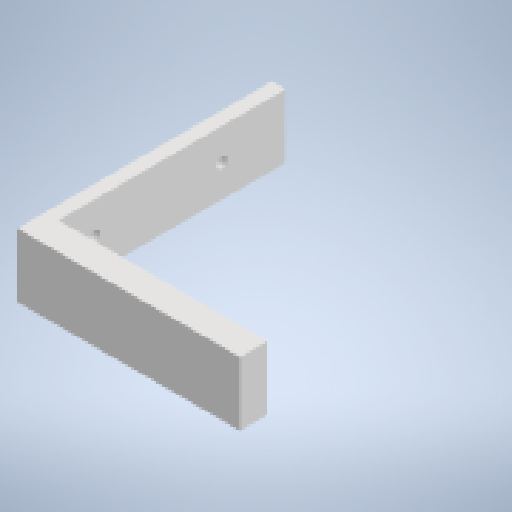
# Autodesk Inventor part: battery shim
Saved by Autodesk Inventor 2023 (Build 270158000, 158)
## iProperties
Created: 2023-02-08
Part Number: battery shim
Material: Generic
Document SubType Name: Modeling
Designer: Gabriel - T3 CAD
Density: 1 g/cm^3
Appearance: Default
Author: Gabriel - T3 CAD
Autodesk Inventor part; units mm, degrees
ref_plane "YZ Plane" through (0, 0, 0) normal (1, 0, 0) x (0, 1, 0)
ref_plane "XZ Plane" through (0, 0, 0) normal (0, 1, 0) x (-1, 0, 0)
ref_plane "XY Plane" through (0, 0, 0) normal (0, 0, 1) x (1, 0, 0)
sketch "Sketch1" plane through (0, 0, 0) normal (0, 1, 0) x (-1, 0, 0)
  line L0 (0, 0) -> (10.922, 0)
  line L1 (10.922, 0) -> (10.922, 203.2)
  line L2 (10.922, 203.2) -> (0, 203.2)
  line L3 (0, 203.2) -> (0, 0)
  line L4 (10.922, 203.2) -> (-166.878, 203.2)
  line L5 (-166.878, 203.2) -> (-166.878, 181.102)
  line L6 (-166.878, 181.102) -> (10.922, 181.102)
  line L7 (10.922, 181.102) -> (10.922, 203.2)
  point P0 (0, 181.102)
  dimension "d0" = 10.922
  dimension "d1" = 203.2
  dimension "d16" = 177.8
  dimension "d17" = 22.098
  constraints: 16 end point, 4 parallel, 2 horizontal, 2 perpendicular
  measures "d0" distance of L2.end L1.end
  measures "d1" distance of L1.end L0.end
  measures "d16" distance of L6.end L5.end
  measures "d17" distance of L4.end L5.end
extrude "Extrusion1" add sketch "Sketch1" along normal blind 50.8
sketch "Sketch3" plane through (0, 0, 181.102) normal (1, 0, 0) x (0, 0, -1)
  circle A0 centre (28.702, 25.4) radius 2.5797
  circle A1 centre (130.302, 25.4) radius 2.5797
  line L0 (181.102, 0) -> (181.102, 50.8) projected
  line L1 (0, 0) -> (181.102, 0) projected
  circle A2 centre (130.302, 25.4) radius 3.9688
  circle A3 centre (28.702, 25.4) radius 3.9687
  dimension "d18" = 5.1594
  dimension "d19" = 5.1594
  dimension "d20" = 0
  dimension "d21" = 101.6
  dimension "d22" = 50.8
  dimension "d23" = 25.4
  dimension "d24" = 7.9375
  dimension "d25" = 7.9375
  constraints: 4 centre point, 2 coincident
  measures "d18" diameter of A1
  measures "d19" diameter of A0
  measures "d20" vertical distance of A1.centre A0.centre
  measures "d21" distance of A0.centre A1.centre
  measures "d22" distance from line of L0 A1.centre
  measures "d23" distance from line of L1 A0.centre
  measures "d24" diameter of A2
  measures "d25" diameter of A3
sketch "Sketch4" plane through (166.878, 0, 181.102) normal (0, 0, -1) x (-1, 0, 0)
  circle A0 centre (50.8, 25.4) radius 2.5797
  circle A1 centre (127, 25.4) radius 2.5797
  line L0 (0, 0) -> (0, 50.8) projected
  circle A2 centre (50.8, 25.4) radius 3.9687
  circle A3 centre (127, 25.4) radius 3.9687
  line L1 (0, 0) -> (166.878, 0) projected
  dimension "d26" = 5.1594
  dimension "d27" = 5.1594
  dimension "d28" = 0
  dimension "d29" = 76.2
  dimension "d30" = 50.8
  dimension "d31" = 7.9375
  dimension "d32" = 7.9375
  dimension "d33" = 25.4
  constraints: 4 centre point, 2 coincident
  measures "d26" diameter of A1
  measures "d27" diameter of A0
  measures "d28" vertical distance of A0.centre A1.centre
  measures "d29" distance of A0.centre A1.centre
  measures "d30" distance from line of L0 A0.centre
  measures "d31" diameter of A3
  measures "d32" diameter of A2
  measures "d33" distance from line of L1 A0.centre
extrude "Extrusion4" cut sketch "Sketch4" against normal through all contours A0 | A1
extrude "Extrusion5" cut sketch "Sketch4" against normal blind 5.1594 contours A0 | A1 | A2 | A3
extrude "Extrusion6" cut sketch "Sketch3" against normal blind 5.1594 contours A0 | A1 | A2 | A3
extrude "Extrusion7" cut sketch "Sketch3" against normal through all contours A0 | A1
equation "\"d19\" = d18"
equation "\"d26\" = d18"
equation "\"d27\" = d26"
equation "\"d31\" = d24"
equation "\"d32\" = d31"
body "Solid1"
